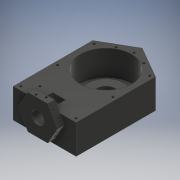
# Autodesk Inventor part: AC01
Saved by Autodesk Inventor 2017 (Build 210142000, 142)
## iProperties
Created: 2019-08-28
Part Number: AC01
Material: ABS Plastic
Document SubType Name: Modeling
Designer: Dell
Density: 1.06 g/cm^3
Appearance: Smooth - Black
Mass: 650.068 g
Surface Area: 1285.03 cm^2
Volume: 613.271 cm^3
Author: Dell
Autodesk Inventor part; units mm, degrees
ref_plane "YZ Plane" through (0, 0, 0) normal (1, 0, 0) x (0, 1, 0)
ref_plane "XZ Plane" through (0, 0, 0) normal (0, 1, 0) x (-1, 0, 0)
ref_plane "XY Plane" through (0, 0, 0) normal (0, 0, 1) x (1, 0, 0)
sketch "Sketch1" plane through (0, 0, 0) normal (0, 0, 1) x (1, 0, 0)
  circle A0 centre (0, 0) radius 17.5
  circle A1 centre (0, 0) radius 67.5
  circle A2 centre (41.5, 0) radius 2
  circle A3 centre (29.3449, 29.3449) radius 2
  circle A4 centre (0, 41.5) radius 2
  circle A5 centre (-29.3449, 29.3449) radius 2
  circle A6 centre (-41.5, 0) radius 2
  circle A7 centre (-29.3449, -29.3449) radius 2
  circle A8 centre (0, -41.5) radius 2
  circle A9 centre (29.3449, -29.3449) radius 2
  dimension "d0" = 35
  dimension "d1" = 135
  dimension "d2" = 4
  dimension "d3" = 41.5
  dimension "d6" = 360
  constraints: 10 centre point, 2 coincident, 1 horizontal alignment, 17 other
  measures "d0" diameter of A0
  measures "d1" diameter of A1
  measures "d2" diameter of A2
  measures "d3" distance of A2.centre point (0, 0)
extrude "Extrusion1" add sketch "Sketch1" along normal blind 15
sketch "Sketch5" plane through (0, 0, 15) normal (0, 0, 1) x (1, 0, 0)
  circle A0 centre (0, 0) radius 67.5 projected
  circle A1 centre (0, 0) radius 48.5
  dimension "d19" = 97
  constraints: 1 centre point
  measures "d19" diameter of A1
extrude "Extrusion4" add sketch "Sketch5" along normal blind 40
sketch "Sketch11" plane through (0, 0, 55) normal (0, 0, 1) x (1, 0, 0)
  line L0 (0, 77.9423) -> (67.5, 38.9711)
  line L1 (67.5, 38.9711) -> (67.5, -38.9711)
  line L2 (67.5, -38.9711) -> (0, -77.9423)
  line L3 (0, -77.9423) -> (-67.5, -38.9711)
  line L4 (-67.5, -38.9711) -> (-67.5, 38.9711)
  line L5 (-67.5, 38.9711) -> (0, 77.9423)
  circle A0 centre (0, 0) radius 67.5 projected
  constraints: 12 end point, 1 coincident, 1 tangent, 1 vertical alignment, 13 other
extrude "Extrusion8" add sketch "Sketch11" against normal blind 55 contours L0 A0 L5 | L0 L1 A0 | A0 L4 L5 | L1 L2 A0 | A0 L3 L4 | L2 L3 A0
sketch "Sketch16" plane through (0, 0, 15) normal (0, 0, 1) x (1, 0, 0)
  circle A0 centre (-41.5, 0) radius 2 projected
  circle A1 centre (0, 0) radius 34.5
  circle A2 centre (0, 0) radius 48.5
  line L0 (-48.5, 0) -> (-34.5, 0)
  circle A3 centre (0, 0) radius 48.5 projected
  constraints: 3 coincident, 3 horizontal alignment, 2 end point, 1 horizontal, 1 midpoint, 5 other
extrude "Extrusion11" cut sketch "Sketch16" against normal blind 8
sketch "Sketch19" plane through (0, 0, 55) normal (0, 0, 1) x (1, 0, 0)
  circle A0 centre (0, 0) radius 48.5 projected
  line L0 (0, -77.9423) -> (-67.5, -38.9711) projected
  line L1 (67.5, -38.9711) -> (0, -77.9423) projected
  line L2 (67.5, 38.9711) -> (67.5, -38.9711) projected
  line L3 (0, 77.9423) -> (67.5, 38.9711) projected
  line L4 (-67.5, 38.9711) -> (0, 77.9423) projected
  line L5 (-67.5, -38.9711) -> (-67.5, 38.9711) projected
  line L6 (0, 68.1273) -> (59, 34.0637)
  line L7 (59, 34.0637) -> (59, -34.0637)
  line L8 (59, -34.0637) -> (0, -68.1273)
  line L9 (0, -68.1273) -> (-59, -34.0637)
  line L10 (-59, -34.0637) -> (-59, 34.0637)
  line L11 (-59, 34.0637) -> (0, 68.1273)
  dimension "d58" = 118
  constraints: 12 end point, 5 other
  measures "d58" distance between parallel lines of L7 L10
extrude "Extrusion13" cut sketch "Sketch19" against normal through all contours L0 L5 L4 L3 L2 L1
sketch "Sketch20" plane through (0, 0, 0) normal (0, 0, -1) x (-1, 0, 0)
  line L0 (-59, -34.0637) -> (-59, -115)
  line L1 (-59, -115) -> (59, -115)
  line L2 (59, -34.0637) -> (59, 34.0637) projected
  line L3 (59, -115) -> (59, -34.0637)
  line L4 (-59, -34.0637) -> (0, -68.1273) projected
  line L5 (0, -68.1273) -> (59, -34.0637) projected
  line L6 (-59, -34.0637) -> (0, -68.1273)
  line L7 (0, -68.1273) -> (59, -34.0637)
  point P0 (0, 0)
  dimension "d61" = 115
  constraints: 10 end point, 2 vertical, 1 collinear, 1 horizontal
  measures "d61" distance from line of point (0, 0) L1
extrude "Extrusion14" add sketch "Sketch20" against normal blind 55
sketch "Sketch22" plane through (0, 0, 55) normal (0, 0, 1) x (1, 0, 0)
  line L0 (59, -115) -> (59, 34.0637) construction
  line L1 (59, 34.0637) -> (0, 68.1273) construction
  line L2 (0, 68.1273) -> (-59, 34.0637) construction
  line L3 (-59, 34.0637) -> (-59, -115) construction
  line L4 (-59, -115) -> (59, -115) construction
  line L5 (52, 30.0222) -> (52, -108) construction
  line L6 (52, -108) -> (-52, -108) construction
  line L7 (-52, -108) -> (-52, 30.0222) construction
  line L8 (-52, 30.0222) -> (0, 60.0444) construction
  line L9 (0, 60.0444) -> (52, 30.0222) construction
  circle A0 centre (-52, -108) radius 2
  circle A1 centre (52, -108) radius 2
  circle A2 centre (0, 60.0444) radius 2
  circle A3 centre (-52, 30.0222) radius 2
  circle A4 centre (52, 30.0222) radius 2
  circle A5 centre (-26, -108) radius 2
  circle A6 centre (26, -108) radius 2
  circle A7 centre (0, -108) radius 2
  circle A8 centre (-52, -68.9889) radius 2
  circle A9 centre (-52, -38.9889) radius 2
  circle A10 centre (-52, 0) radius 2
  circle A11 centre (52, 0) radius 2
  circle A12 centre (52, -38.9889) radius 2
  circle A13 centre (52, -68.9889) radius 2
  circle A14 centre (-26, 45.0333) radius 2
  circle A15 centre (26, 45.0333) radius 2
  point P0 (0, 0)
  point P1 (0, 0)
  point P2 (0, 68.1273)
  point P3 (59, 34.0637)
  dimension "d64" = 7
  dimension "d65" = 4
  dimension "d66" = 4
  dimension "d67" = 4
  dimension "d68" = 4
  dimension "d69" = 4
  dimension "d70" = 4
  dimension "d71" = 4
  dimension "d72" = 4
  dimension "d73" = 4
  dimension "d74" = 4
  dimension "d75" = 4
  dimension "d76" = 4
  dimension "d77" = 4
  dimension "d78" = 4
  dimension "d79" = 4
  dimension "d80" = 4
  dimension "d81" = 30
  constraints: 20 end point, 16 centre point, 11 coincident, 6 point on line, 5 midpoint, 3 horizontal alignment, 2 vertical alignment, 4 other
  measures "d64" distance between parallel lines of L0 L5
  measures "d65" diameter of A0
  measures "d66" diameter of A1
  measures "d67" diameter of A2
  measures "d68" diameter of A3
  measures "d69" diameter of A4
  measures "d70" diameter of A5
  measures "d71" diameter of A6
  measures "d72" diameter of A7
  measures "d73" diameter of A8
  measures "d74" diameter of A9
  measures "d75" diameter of A10
  measures "d76" diameter of A11
  measures "d77" diameter of A12
  measures "d78" diameter of A13
  measures "d79" diameter of A14
  measures "d80" diameter of A15
  measures "d81" distance of A9.centre A8.centre
extrude "Extrusion15" cut sketch "Sketch22" against normal through all contours A0 | A1 | A3 | A4 | A9 | A12 | A14 | A15
sketch "Sketch23" plane through (-59, -115, 0) normal (0, -1, 0) x (1, 0, 0)
  line L0 (12.812, 40) -> (35.906, 80)
  line L1 (35.906, 80) -> (82.094, 80)
  line L2 (82.094, 80) -> (105.188, 40)
  line L3 (105.188, 40) -> (82.094, 0)
  line L4 (82.094, 0) -> (35.906, 0)
  line L5 (35.906, 0) -> (12.812, 40)
  line L6 (118, 0) -> (0, 0) projected
  point P0 (59, 0)
  point P1 (59, 40)
  point P2 (59, 0)
  point P3 (59, 0)
  dimension "d87" = 80
  constraints: 12 end point, 3 midpoint, 1 horizontal, 1 vertical alignment, 13 other
  measures "d87" distance between parallel lines of L1 L4
extrude "Extrusion16" add sketch "Sketch23" along normal blind 13
sketch "Sketch24" plane through (-59, -128, 0) normal (0, -1, 0) x (1, 0, 0)
  line L0 (35.906, 80) -> (12.812, 40) projected
  line L1 (12.812, 40) -> (35.906, 0) projected
  line L2 (35.906, 0) -> (82.094, 0) projected
  line L3 (82.094, 0) -> (105.188, 40) projected
  line L4 (105.188, 40) -> (82.094, 80) projected
  line L5 (82.094, 80) -> (35.906, 80) projected
  line L6 (40.5248, 8) -> (22.0496, 40)
  line L7 (22.0496, 40) -> (40.5248, 72)
  line L8 (40.5248, 72) -> (77.4752, 72)
  line L9 (77.4752, 72) -> (95.9504, 40)
  line L10 (95.9504, 40) -> (77.4752, 8)
  line L11 (77.4752, 8) -> (40.5248, 8)
  point P0 (59, 0)
  dimension "d88" = 8
  constraints: 12 end point, 5 other
  measures "d88" distance between parallel lines of L1 L6
extrude "Extrusion17" cut sketch "Sketch24" against normal up to surface (13 mm away) from surface at 0
sketch "Sketch25" plane through (-59, -128, 0) normal (0, -1, 0) x (1, 0, 0)
  line L0 (95.9504, 40) -> (77.4752, 72) projected
  line L1 (77.4752, 72) -> (40.5248, 72) projected
  line L2 (40.5248, 72) -> (22.0496, 40) projected
  line L3 (22.0496, 40) -> (40.5248, 8) projected
  line L4 (40.5248, 8) -> (77.4752, 8) projected
  line L5 (77.4752, 8) -> (95.9504, 40) projected
  circle A0 centre (59, 40) radius 12
  point P0 (59, 0)
  point P1 (59, 72)
  dimension "d91" = 24
  constraints: 1 centre point, 1 horizontal alignment, 1 midpoint, 1 vertical alignment
  measures "d91" diameter of A0
extrude "Extrusion18" cut sketch "Sketch25" against normal blind 40 contours A0
sketch "Sketch26" plane through (0, 0, 55) normal (0, 0, 1) x (1, 0, 0)
  line L0 (12, -88) -> (-12, -88) projected
  line L1 (12, -128) -> (-12, -128) projected
  line L2 (12, -88) -> (-12, -88) projected
  line L3 (-12, -88) -> (12, -88)
  line L4 (12, -88) -> (12, -101)
  line L5 (12, -101) -> (-12, -101)
  line L6 (-12, -101) -> (-12, -88)
  point P0 (0, 0)
  dimension "d94" = 13
  constraints: 8 end point, 2 parallel, 1 horizontal, 1 perpendicular
  measures "d94" distance between parallel lines of L0 L5
extrude "Extrusion19" cut sketch "Sketch26" against normal blind 15
sketch "Sketch27" plane through (-36.9504, -128, 40) normal (-0.866, 0, 0.5) x (0.5, 0, 0.866)
  line L0 (17.3205, 13) -> (36.9504, 13) projected
  line L1 (17.3205, 13) -> (0, 13) projected
  line L2 (0, 0) -> (0, 13) projected
  line L3 (36.9504, 0) -> (0, 0) projected
  line L4 (36.9504, 0) -> (36.9504, 13) projected
  circle A0 centre (11.4041, 4) radius 2
  circle A1 centre (25.5463, 9) radius 2
  line L5 (11.4041, 4) -> (25.5463, 9) construction
  line L6 (0, 13) -> (36.9504, 13) projected
  point P0 (-16.1658, 128)
  point P1 (18.4752, 6.5)
  point P2 (18.4752, 13)
  point P3 (0, 6.5)
  dimension "d97" = 4
  dimension "d98" = 4
  dimension "d99" = 15
  dimension "d112" = 5
  constraints: 3 midpoint, 2 centre point, 2 end point, 1 horizontal alignment, 1 vertical alignment
  measures "d97" diameter of A0
  measures "d98" diameter of A1
  measures "d99" distance of L5.start L5.end
  measures "d112" vertical distance of L5.end L5.start
extrude "Extrusion20" cut sketch "Sketch27" against normal blind 20 contours A0 | A1
pattern_circular "Circular Pattern1" count 6 over 360 about axis through (0, -128, 40) along (0, 1, 0) of "Extrusion20"
sketch "Sketch28" plane through (0, 0, 55) normal (0, 0, 1) x (1, 0, 0)
  circle A0 centre (0, 53.1273) radius 2
  circle A1 centre (-34, -90) radius 2
  line L0 (-59, 34.0637) -> (-59, -115) projected
  line L1 (-59, -115) -> (-28.2902, -115) projected
  point P0 (0, 0)
  point P1 (0, 68.1273)
  dimension "d105" = 4
  dimension "d106" = 15
  dimension "d107" = 4
  dimension "d108" = 25
  dimension "d109" = 25
  constraints: 2 centre point, 1 vertical alignment
  measures "d105" diameter of A0
  measures "d106" distance of A0.centre point (0, 68.127)
  measures "d107" diameter of A1
  measures "d108" distance from line of L0 A1.centre
  measures "d109" distance from line of L1 A1.centre
extrude "Extrusion21" cut sketch "Sketch28" against normal through all
sketch "Sketch30" plane through (0, 0, 55) normal (0, 0, 1) x (1, 0, 0)
  circle A0 centre (0, 0) radius 48.5 construction
  line L0 (12, -88) -> (12, -101) construction
  line L1 (12, -88) -> (-12, -88) construction
  line L2 (-12, -88) -> (-12, -101) construction
  line L3 (-12, -101) -> (12, -101) construction
  line L4 (12, -128) -> (-12, -128) construction
  circle A1 centre (-34, -90) radius 2 construction
  line L5 (-17, -83) -> (17, -83) construction
  line L6 (17, -83) -> (17, -106) construction
  line L7 (17, -106) -> (-17, -106) construction
  line L8 (-17, -106) -> (-17, -83) construction
  circle A2 centre (-34, -90) radius 7 construction
  circle A3 centre (0, 0) radius 53.5 construction
  circle A4 centre (0, 53.1273) radius 2 construction
  circle A5 centre (-34, -90) radius 2 construction
  line L9 (-12, -101) -> (-12, -88) construction
  line L10 (-12, -88) -> (12, -88) construction
  line L11 (12, -88) -> (12, -101) construction
  line L12 (12, -101) -> (-12, -101) construction
  circle A6 centre (26, 45.0333) radius 2 construction
  circle A7 centre (-52, 30.0222) radius 2 construction
  circle A8 centre (-52, -108) radius 2 construction
  circle A9 centre (52, -38.9889) radius 2 construction
  circle A10 centre (52, -108) radius 2 construction
  circle A11 centre (-52, -38.9889) radius 2 construction
  circle A12 centre (-26, 45.0333) radius 2 construction
  circle A13 centre (52, 30.0222) radius 2 construction
  line L13 (0, 68.1273) -> (-59, 34.0637) construction
  line L14 (-59, 34.0637) -> (-59, -115) construction
  line L15 (-59, -115) -> (-28.2902, -115) construction
  line L16 (-28.2902, -115) -> (28.2902, -115) construction
  line L17 (28.2902, -115) -> (59, -115) construction
  line L18 (59, -115) -> (59, 34.0637) construction
  line L19 (59, 34.0637) -> (0, 68.1273) construction
  circle A14 centre (0, 0) radius 48.5 construction
  line L20 (-46, -102) -> (-46, 26.5581) construction
  line L21 (-46, 26.5581) -> (0, 53.1162) construction
  line L22 (0, 53.1162) -> (46, 26.5581) construction
  line L23 (46, 26.5581) -> (46, -102) construction
  line L24 (46, -102) -> (28.2902, -102) construction
  line L25 (28.2902, -102) -> (-28.2902, -102) construction
  line L26 (-28.2902, -102) -> (-46, -102) construction
  line L27 (-23, -50.9295) -> (-8, -59.5897)
  line L28 (-8, -59.5897) -> (-8, -76.9103)
  line L29 (-8, -76.9103) -> (-23, -85.5705)
  line L30 (-23, -85.5705) -> (-38, -76.9103)
  line L31 (-38, -76.9103) -> (-38, -59.5897)
  line L32 (-38, -59.5897) -> (-23, -50.9295)
  line L33 (23, -50.9295) -> (38, -59.5897)
  line L34 (38, -59.5897) -> (38, -76.9103)
  line L35 (38, -76.9103) -> (23, -85.5705)
  line L36 (23, -85.5705) -> (8, -76.9103)
  line L37 (8, -76.9103) -> (8, -59.5897)
  line L38 (8, -59.5897) -> (23, -50.9295)
  line L39 (0, -83) -> (-46, -83) construction
  line L40 (0, -83) -> (46, -83) construction
  line L41 (0, -53.5) -> (0, -83) construction
  point P0 (-23, -68.25)
  point P1 (23, -68.25)
  point P2 (-23, -83)
  point P3 (23, -83)
  point P4 (0, -68.25)
  dimension "d121" = 5
  dimension "d122" = 5
  dimension "d123" = 5
  dimension "d124" = 13
  dimension "d125" = 30
  constraints: 52 end point, 5 vertical alignment, 4 midpoint, 3 horizontal alignment, 3 point on line, 2 vertical, 1 centre point, 1 perpendicular, 37 other
  measures "d121" distance between parallel lines of L1 L5
  measures "d122" radial gap between concentric circles of A1 A2
  measures "d124" distance between parallel lines of L14 L20
  measures "d125" distance between parallel lines of L34 L37
extrude "Extrusion23" [suppressed]
sketch "Sketch31" plane through (0, 0, 5) normal (0, 0, 1) x (1, 0, 0)
  line L0 (-52.3536, -52.747) -> (-52.3536, -97.747)
  line L1 (-52.3536, -97.747) -> (-41.747, -108.3536)
  line L2 (-41.747, -108.3536) -> (-26.747, -108.3536)
  circle A0 centre (-52, -108) radius 2 projected
  line L3 (-52, -108) -> (-47.0503, -103.0503)
  line L4 (-26.747, -98.3536) -> (-37.6048, -98.3536)
  line L5 (-37.6048, -98.3536) -> (-42.3536, -93.6048)
  line L6 (-42.3536, -93.6048) -> (-42.3536, -52.747)
  line L7 (-52.3536, -52.747) -> (-42.3536, -52.747)
  line L8 (-26.747, -98.3536) -> (-26.747, -108.3536)
  point P0 (0, 0)
  dimension "d128" = 45
  dimension "d129" = 15
  dimension "d130" = 15
  dimension "d131" = 135
  dimension "d132" = 7
  dimension "d133" = 10
  constraints: 18 end point, 4 perpendicular, 1 horizontal, 1 midpoint, 1 vertical, 2 other
  measures "d128" distance of L0.start L0.end
  measures "d129" distance of L1.end L2.end
  measures "d130" distance of L0.end L1.end
  measures "d131" angle of L0 L1
  measures "d132" distance of L3.start L3.end
  measures "d133" distance between parallel lines of L1 L5
extrude "Extrusion24" [suppressed]
mirror "Mirror1" [suppressed]
sketch "Sketch32" plane through (0, 0, 0) normal (0, 0, -1) x (-1, 0, 0)
  circle A0 centre (0, 0) radius 33
  dimension "d139" = 66
  constraints: 1 centre point, 1 coincident
  measures "d139" diameter of A0
extrude "Extrusion25" cut sketch "Sketch32" against normal blind 2
body "Solid1"
